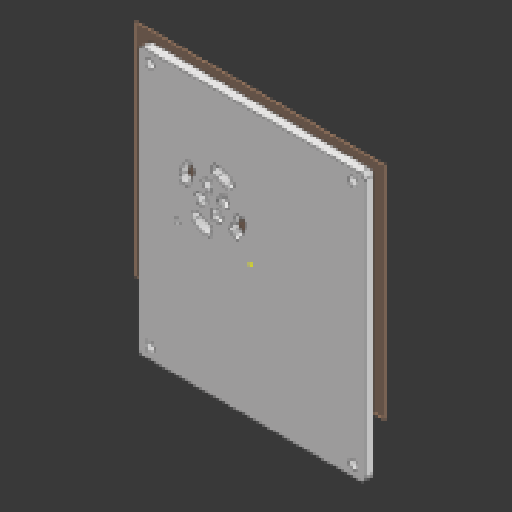
# Autodesk Inventor part: Picover
Saved by Autodesk Inventor 2023 (Build 270158000, 158)
## iProperties
Created: 2022-12-29
Part Number: Picover
Material: Generic
Document SubType Name: Modeling
Designer: alber
Density: 1 g/cm^3
Appearance: Default
Author: alber
Autodesk Inventor part; units mm, degrees
ref_plane "YZ Plane" through (0, 0, 0) normal (1, 0, 0) x (0, 1, 0)
ref_plane "XZ Plane" through (0, 0, 0) normal (0, 1, 0) x (-1, 0, 0)
ref_plane "XY Plane" through (0, 0, 0) normal (0, 0, 1) x (1, 0, 0)
ref_plane "Work Plane1" through (0, 0, 0) normal (0, 0, 1) x (1, 0, 0)
sketch "Sketch2" plane through (0, 0, 0) normal (0, 0, 1) x (1, 0, 0)
  line L0 (-50.7403, -58) -> (-50.7403, -45) projected
  line L1 (50.7403, 58) -> (50.7403, 44) projected
  line L2 (-50.7403, -58) -> (-50.7403, -45) projected
  arc A0 (-47.4372, -45) -> (-35.7403, -56.6969) centre (-32.7403, -42) ccw projected
  circle A1 centre (-45.7403, -55) radius 2 projected
  line L3 (-50.7403, -60) -> (50.7403, -60)
  line L4 (50.7403, -60) -> (50.7403, 60)
  line L5 (50.7403, 60) -> (-50.7403, 60)
  line L6 (-50.7403, 60) -> (-50.7403, -60)
  line L7 (-40.7403, -60) -> (-20.7403, -60)
  line L8 (-20.7403, -60) -> (-20.7403, -55)
  line L9 (-20.7403, -55) -> (-40.7403, -55)
  line L10 (-40.7403, -55) -> (-40.7403, -60)
  line L11 (50.7403, -32) -> (45.7403, -32)
  line L12 (45.7403, -32) -> (45.7403, 44)
  line L13 (45.7403, 44) -> (50.7403, 44)
  line L14 (50.7403, 44) -> (50.7403, -32)
  line L15 (-50.7403, -50) -> (-45.7403, -50)
  line L16 (-45.7403, -50) -> (-45.7403, -30.0278)
  line L17 (-45.7403, -30.0278) -> (-50.7403, -30.0278)
  line L18 (-50.7403, -30.0278) -> (-50.7403, -50)
  arc A2 (-47.4372, -45) -> (-35.7403, -56.6969) centre (-32.7403, -42) ccw projected
  circle A3 centre (-45.7403, -55) radius 2 projected
  circle A4 centre (-45.7403, 55) radius 2 projected
  circle A5 centre (45.7403, 55) radius 2 projected
  arc A6 (50.7403, 58) -> (48.7403, 60) centre (48.7403, 58) ccw projected
  line L19 (-48.7403, 60) -> (48.7403, 60) projected
  arc A7 (-48.7403, 60) -> (-50.7403, 58) centre (-48.7403, 58) ccw projected
  line L20 (-50.7403, -19) -> (-50.7403, 58) projected
  line L21 (-47.7403, 42) -> (-47.7403, -19) projected
  arc A8 (-32.7403, 57) -> (-47.7403, 42) centre (-32.7403, 42) ccw projected
  line L22 (32.7403, 57) -> (-32.7403, 57) projected
  arc A9 (47.6064, 44) -> (32.7403, 57) centre (32.7403, 42) ccw projected
  line L23 (50.7403, 44) -> (47.6064, 44) projected
  circle A10 centre (45.7403, -55) radius 2 projected
  line L24 (-35.7403, -60) -> (-48.7403, -60) projected
  line L25 (-35.7403, -56.6969) -> (-35.7403, -60) projected
  line L26 (-50.7403, -45) -> (-47.4372, -45) projected
  line L27 (-35.7403, -60) -> (-48.7403, -60) projected
  line L28 (-35.7403, -56.6969) -> (-35.7403, -60) projected
  line L29 (-50.7403, -45) -> (-47.4372, -45) projected
  line L30 (-47.7403, -19) -> (-50.7403, -19) projected
  arc A11 (-50.7403, -58) -> (-48.7403, -60) centre (-48.7403, -58) ccw projected
  arc A12 (-50.7403, -58) -> (-48.7403, -60) centre (-48.7403, -58) ccw projected
  point P0 (0, 0)
  point P1 (-47.7403, -50)
  point P2 (-40.7403, -57)
  point P3 (50.7403, 44)
  point P4 (-50.7403, -30)
  dimension "d0" = 5
  dimension "d1" = 5
  dimension "d2" = 5
  constraints: 32 end point, 8 parallel, 4 horizontal, 4 perpendicular
  measures "d0" distance of L8.end L7.end
  measures "d1" distance of L12.end L13.end
  measures "d2" distance of L17.end L16.end
extrude "Extrusion1" add sketch "Sketch2" along normal blind 4
fillet "Fillet1" radius 2 2 edges at (50.7403, 60, 2) (-50.7403, -60, 2)
sketch "Sketch3" plane through (0, 0, 4) normal (0, 0, 1) x (1, 0, 0)
  circle A0 centre (-33.5708, 0) radius 1.25
  point P0 (0, 0)
  dimension "d6" = 2.5
  constraints: 1 centre point
  measures "d6" diameter of A0
extrude "Extrusion2" cut sketch "Sketch3" against normal blind 15.05
pattern_linear "Rectangular Pattern1" [suppressed]
sketch "Sketch4" plane through (0, 0, 4) normal (0, 0, 1) x (1, 0, 0)
  circle A0 centre (-33.5708, 0) radius 1.25 projected
  circle A1 centre (-1.5708, 0) radius 1.25 projected
  circle A2 centre (-1.5708, 32) radius 1.25 projected
  circle A3 centre (-33.5708, 32) radius 1.25 projected
  circle A4 centre (-33.5708, 0) radius 1.25 projected
  line L0 (-1.5708, 32) -> (-33.5708, 32)
  line L1 (-33.5708, 32) -> (-33.5708, 0)
  line L2 (-33.5708, 0) -> (-1.5708, 0)
  line L3 (-1.5708, 0) -> (-1.5708, 32)
  circle A5 centre (-17.5708, 16) radius 15
  circle A6 centre (-17.5708, 16) radius 10
  circle A7 centre (-17.5708, 16) radius 7.5
  circle A8 centre (-17.5708, 16) radius 2.5
  circle A9 centre (-1.5708, 0) radius 1.25 projected
  line L4 (-1.5708, 0) -> (-33.5708, 32)
  circle A10 centre (-1.5708, 32) radius 1.25 projected
  line L5 (-33.5708, 0) -> (-1.5708, 32)
  line L6 (-33.5708, 16) -> (-1.5708, 16)
  line L7 (-17.5708, 0) -> (-17.5708, 32)
  point P0 (0, 0)
  point P1 (-17.5708, 18.5)
  point P2 (-17.5708, 23.5)
  point P3 (-22.8741, 21.3033)
  point P4 (-19.3385, 17.7678)
  point P5 (-20.0708, 16)
  point P6 (-25.0708, 16)
  point P7 (-22.8741, 10.6967)
  point P8 (-19.3385, 14.2322)
  point P9 (-17.5708, 13.5)
  point P10 (-17.5708, 8.5)
  point P11 (-12.2674, 10.6967)
  point P12 (-15.803, 14.2322)
  point P13 (-15.0708, 16)
  point P14 (-10.0708, 16)
  point P15 (-12.2674, 21.3033)
  point P16 (-15.803, 17.7678)
  point P17 (-32.5708, 16)
  point P18 (-27.5708, 16)
  point P19 (-24.6418, 23.0711)
  point P20 (-28.1774, 26.6066)
  point P21 (-17.5708, 1)
  point P22 (-17.5708, 6)
  point P23 (-24.6418, 8.9289)
  point P24 (-28.1774, 5.3934)
  point P25 (-2.5708, 16)
  point P26 (-7.5708, 16)
  point P27 (-10.4997, 8.9289)
  point P28 (-6.9641, 5.3934)
  point P29 (-17.5708, 31)
  point P30 (-17.5708, 26)
  point P31 (-10.4997, 23.0711)
  point P32 (-6.9641, 26.6066)
  dimension "d15" = 30
  dimension "d16" = 20
  dimension "d17" = 15
  dimension "d18" = 5
  constraints: 16 end point, 4 centre point, 4 midpoint, 3 coincident, 2 parallel, 2 perpendicular, 1 horizontal
  measures "d15" diameter of A5
  measures "d16" diameter of A6
  measures "d17" diameter of A7
  measures "d18" diameter of A8
extrude "Extrusion3" cut sketch "Sketch4" against normal blind 5.5875 contours L5 A6 L7 A5 | A5 L4 A6 L6 | L4 A6 L6 A5 | A7 L6 A8 L5 | L7 A8 L4 A7 | A5 L5 A6 L7 | A7 L7 A8 L4 | L6 A8 L5 A7
fillet "Fillet2" radius 2 16 edges at (-6.9641, 5.3934, 2) (-10.4997, 8.9289, 2) (-2.5708, 16, 2) (-7.5708, 16, 2) (-28.1774, 5.3934, 2) (-24.6418, 8.9289, 2) (-17.5708, 6, 2) (-17.5708, 1, 2) (-27.5708, 16, 2) (-32.5708, 16, 2) (-24.6418, 23.0711, 2) (-28.1774, 26.6066, 2) (-17.5708, 26, 2) (-17.5708, 31, 2) (-6.9641, 26.6066, 2) (-10.4997, 23.0711, 2)
fillet "Fillet3" radius 1 16 edges at (-12.2674, 10.6967, 2) (-17.5708, 8.5, 2) (-17.5708, 13.5, 2) (-15.803, 14.2322, 2) (-22.8741, 10.6967, 2) (-19.3385, 14.2322, 2) (-20.0708, 16, 2) (-25.0708, 16, 2) (-15.803, 17.7678, 2) (-15.0708, 16, 2) (-10.0708, 16, 2) (-12.2674, 21.3033, 2) (-17.5708, 18.5, 2) (-19.3385, 17.7678, 2) (-22.8741, 21.3033, 2) (-17.5708, 23.5, 2)
sketch "Sketch5" plane through (0, 0, 4) normal (0, 0, 1) x (1, 0, 0)
  point P0 (0, 0)
pattern_linear "Rectangular Pattern2" [suppressed]
fillet "Fillet4" radius 2 2 edges at (-50.7403, 60, 2) (50.7403, -60, 2)
fillet "Fillet5" [suppressed]
sketch "Sketch6" plane through (-48.7403, -60, 0) normal (0, -1, 0) x (1, 0, 0)
  point P0 (48.7403, 0)
sketch "Sketch7" plane through (-48.7403, -60, 0) normal (0, -1, 0) x (1, 0, 0)
  line L0 (16, -37) -> (16, 0) projected
  line L1 (36, -3) -> (36, -7) projected
  line L2 (36.0039, 0) -> (36.0039, 4) projected
  line L3 (16, 0) -> (36.0039, 0)
  line L4 (36.0039, 0) -> (36.0039, 4)
  line L5 (36.0039, 4) -> (16, 4)
  line L6 (16, 4) -> (16, 0)
  point P0 (48.7403, 0)
  constraints: 8 end point, 2 parallel, 1 horizontal, 1 perpendicular, 1 point on line
extrude "Extrusion4" cut sketch "Sketch7" against normal blind 10
sketch "Sketch8" plane through (50.7403, 58, 4) normal (1, 0, 0) x (0, 0, -1)
  line L0 (4, 0) -> (4, -116) projected
  line L1 (0, 0) -> (0, -116) projected
  line L2 (4, -16) -> (0, -16)
  line L3 (0, -16) -> (0, -96)
  line L4 (0, -96) -> (4, -96)
  line L5 (4, -96) -> (4, -16)
  point P0 (4, -58)
  point P1 (6, -96)
  point P2 (6, -16)
  constraints: 8 end point, 2 parallel, 2 point on line, 1 horizontal, 1 perpendicular, 2 other
extrude "Extrusion5" cut sketch "Sketch8" against normal blind 5
sketch "Sketch9" plane through (-50.7403, -58, 0) normal (-1, 0, 0) x (0, 0, 1)
  line L0 (-7, 36) -> (-3, 36) projected
  line L1 (-3, 16) -> (-7, 16) projected
  line L2 (0, 116) -> (0, 0) projected
  line L3 (4, 116) -> (4, 0) projected
  line L4 (0, 36) -> (4, 36)
  line L5 (4, 36) -> (4, 16)
  line L6 (4, 16) -> (0, 16)
  line L7 (0, 16) -> (0, 36)
  point P0 (0, 58)
  point P1 (0, 16)
  constraints: 8 end point, 2 parallel, 2 point on line, 1 horizontal, 1 perpendicular
extrude "Extrusion6" cut sketch "Sketch9" against normal blind 5
fillet "Fillet6" radius 2 12 edges at (-45.7403, -42, 2) (-50.7403, -42, 2) (-45.7403, -22, 2) (-50.7403, -22, 2) (-32.7403, -50, 2) (-32.7403, -60, 2) (-12.7364, -50, 2) (-12.7364, -60, 2) (45.7403, -38, 2) (50.7403, -38, 2) (50.7403, 42, 2) (45.7403, 42, 2)
body "Solid1"
